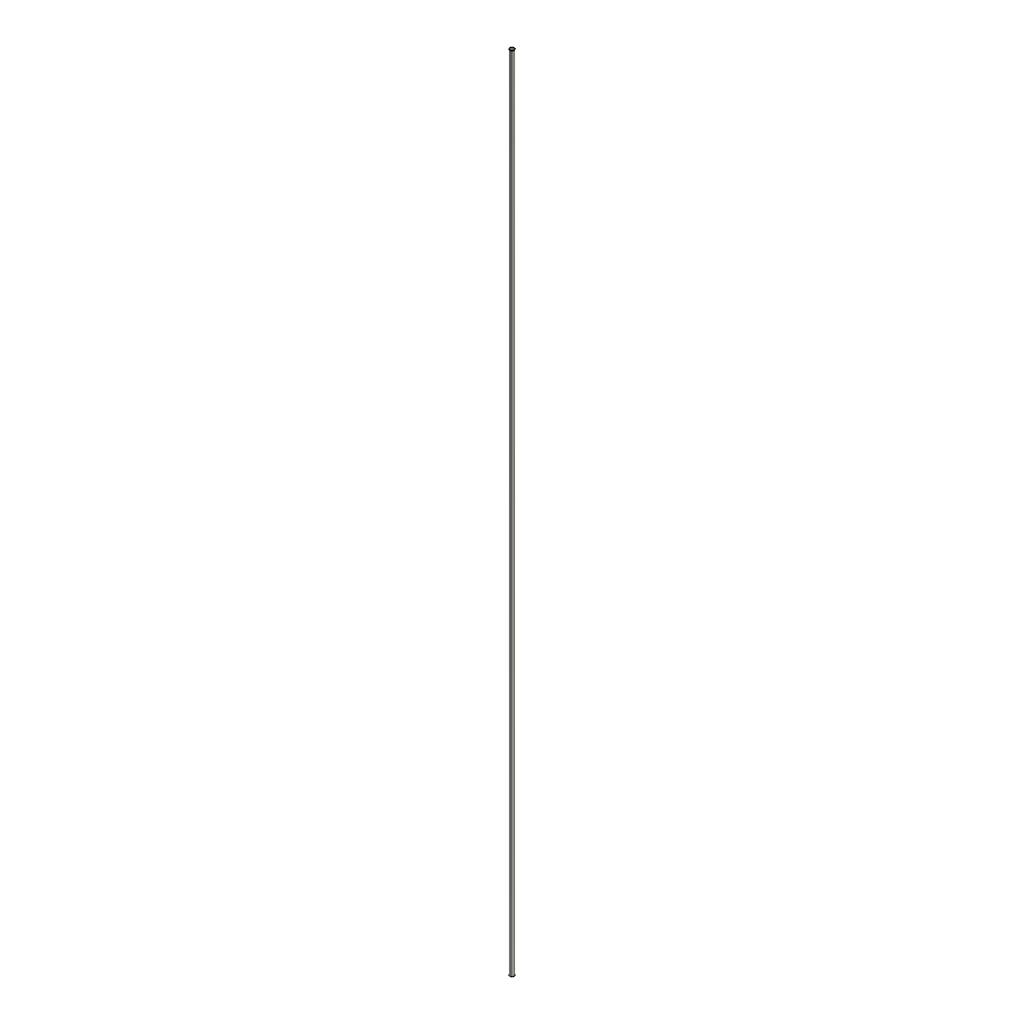
A3_bar (Autodesk Fusion 360 design; units mm, degrees)
part number: 2026-09-10-01-43-12-934
Autodesk Fusion 360 part; units mm, degrees
sketch "Sketch1" plane through (0, 0, 0) normal (0, 0, 1) x (1, 0, 0)
  circle A0 centre (10.16, 12.7) radius 12.7
  dimension "d6" = 25.4
  measures "d6" diameter of A0
extrude "Extrude1" add sketch "Sketch1" along normal blind 4488.5496
equation "Diameter = 1 in"
equation "Load = 400 lbforce"
equation "YoungsModulus = 10000000 psi"
equation "MaxDef = 0.009 in"
equation "Length = ( MaxDef * ( 0.785398 * ( Diameter ^ 2 ) ) * YoungsModulus ) / Load"
equation "d6 = Diameter"
equation "d7 = Length"
